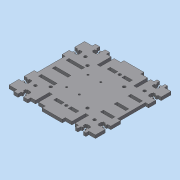
# Autodesk Inventor part: Camera-Holder_Top
Saved by Autodesk Inventor 2016 SP1 (Build 200210100, 210)
## iProperties
Created: 2016-01-28
Part Number: Camera-Holder_Top
Material: Generic
Document SubType Name: Modeling
Designer: Mohamed A.
Density: 1 g/cm^3
Appearance: Default
Author: Mohamed A.
Autodesk Inventor part; units mm, degrees
ref_plane "YZ Plane" through (0, 0, 0) normal (1, 0, 0) x (0, 1, 0)
ref_plane "XZ Plane" through (0, 0, 0) normal (0, 1, 0) x (-1, 0, 0)
ref_plane "XY Plane" through (0, 0, 0) normal (0, 0, 1) x (1, 0, 0)
sketch "Sketch1" plane through (0, 0, 0) normal (0, 0, 1) x (1, 0, 0)
  line L0 (-42.3333, -40) -> (42.3333, -40)
  line L1 (42.3333, -40) -> (42.3333, 40)
  line L2 (42.3333, 40) -> (-42.3333, 40)
  line L3 (-42.3333, 40) -> (-42.3333, -40)
  line L4 (0, 40) -> (0, -40) construction
  line L5 (42.3333, 0) -> (-42.3333, 0) construction
  point P0 (0, 0)
  dimension "d0" = 84.6667
  dimension "d1" = 80
  constraints: 12 end point, 6 midpoint, 2 parallel, 1 horizontal, 1 perpendicular
  measures "d0" distance of L2.end L1.end
  measures "d1" distance of L1.end L0.end
extrude "Extrusion1" add sketch "Sketch1" along normal blind 3
sketch "Sketch2" plane through (-42.3333, 40, 0) normal (0, 1, 0) x (1, 0, 0)
  line L0 (26, -3) -> (26, 0)
  line L1 (26, 0) -> (29, 0)
  line L2 (29, 0) -> (29, -3)
  line L3 (29, -30) -> (26, -30)
  line L4 (0, -3) -> (0, 0)
  line L5 (0, 0) -> (3, 0)
  line L6 (3, 0) -> (3, -3)
  line L7 (3, -30) -> (0, -30)
  line L8 (61.6667, -3) -> (61.6667, 0)
  line L9 (61.6667, 0) -> (64.6667, 0)
  line L10 (64.6667, 0) -> (64.6667, -3)
  line L11 (64.6667, -30) -> (61.6667, -30)
  line L12 (81.6667, -3) -> (81.6667, 0)
  line L13 (81.6667, 0) -> (84.6667, 0)
  line L14 (84.6667, 0) -> (84.6667, -3)
  line L15 (84.6667, -30) -> (81.6667, -30)
  line L16 (84.6667, -3) -> (0, -3) projected
  line L17 (0, -3) -> (3, -3)
  line L18 (26, -3) -> (29, -3)
  line L19 (0, 0) -> (84.6667, 0) projected
  line L20 (3, -3) -> (7.6, -3)
  line L21 (7.6, -3) -> (7.6, 0)
  line L22 (7.6, 0) -> (3, 0)
  line L23 (3, 0) -> (3, -3)
  line L24 (26, -3) -> (21.4, -3)
  line L25 (21.4, -3) -> (21.4, 0)
  line L26 (21.4, 0) -> (26, 0)
  line L27 (26, 0) -> (26, -3)
  line L28 (29, -3) -> (35.5333, -3)
  line L29 (35.5333, -3) -> (35.5333, 0)
  line L30 (35.5333, 0) -> (29, 0)
  line L31 (29, 0) -> (29, -3)
  line L32 (61.6667, -3) -> (55.1333, -3)
  line L33 (55.1333, -3) -> (55.1333, 0)
  line L34 (55.1333, 0) -> (61.6667, 0)
  line L35 (61.6667, 0) -> (61.6667, -3)
  line L36 (64.6667, -3) -> (68.0667, -3)
  line L37 (68.0667, -3) -> (68.0667, 0)
  line L38 (68.0667, 0) -> (64.6667, 0)
  line L39 (64.6667, 0) -> (64.6667, -3)
  line L40 (81.6667, -3) -> (78.2667, -3)
  line L41 (78.2667, -3) -> (78.2667, 0)
  line L42 (78.2667, 0) -> (81.6667, 0)
  line L43 (81.6667, 0) -> (81.6667, -3)
  line L44 (81.6667, -3) -> (84.6667, -3)
  line L45 (64.6667, -3) -> (61.6667, -3)
  line L46 (29, -3) -> (26, -3)
  point P0 (42.3333, 0)
  dimension "d6" = 23
  dimension "d7" = 4.6
  dimension "d8" = 4.6
  dimension "d9" = 17
  dimension "d10" = 3.4
  dimension "d11" = 3.4
  dimension "d12" = 32.6667
  dimension "d34" = 6.5333
  dimension "d35" = 6.5333
  constraints: 90 end point, 14 horizontal, 12 parallel, 8 point on line, 8 vertical, 6 perpendicular, 3 collinear, 23 other
  measures "d6" distance between parallel lines of L23 L27
  measures "d7" distance between parallel lines of L25 L27
  measures "d8" distance between parallel lines of L23 L21
  measures "d9" distance between parallel lines of L10 L12
  measures "d10" distance between parallel lines of L41 L12
  measures "d11" distance between parallel lines of L10 L37
  measures "d12" distance between parallel lines of L31 L8
  measures "d34" distance between parallel lines of L31 L29
  measures "d35" distance between parallel lines of L33 L35
extrude "Extrusion2" cut sketch "Sketch2" against normal blind 3 contours L16 L25 L19 L0 | L0 L1 L2 L16 | L2 L19 L29 L16 | L16 L6 L19 L21 | L33 L19 L8 L16 | L16 L4 L5 L6 | L8 L9 L10 L16 | L10 L19 L37 L16 | L41 L19 L12 L16 | L12 L13 L14 L16
sketch "Sketch3" plane through (-42.3333, -40, 0) normal (0, -1, 0) x (1, 0, 0)
  line L0 (21.4, 3) -> (21.4, 0) projected
  line L1 (35.5333, 0) -> (35.5333, 3) projected
  line L2 (21.4, 0) -> (35.5333, 0) projected
  line L3 (35.5333, 3) -> (21.4, 3) projected
  line L4 (7.6, 0) -> (7.6, 3) projected
  line L5 (0, 0) -> (7.6, 0) projected
  line L6 (0, 3) -> (0, 0) projected
  line L7 (7.6, 3) -> (0, 3) projected
  line L8 (84.6667, 0) -> (84.6667, 3) projected
  line L9 (78.2667, 0) -> (84.6667, 0) projected
  line L10 (78.2667, 3) -> (78.2667, 0) projected
  line L11 (84.6667, 3) -> (78.2667, 3) projected
  line L12 (68.0667, 0) -> (68.0667, 3) projected
  line L13 (55.1333, 0) -> (68.0667, 0) projected
  line L14 (55.1333, 3) -> (55.1333, 0) projected
  line L15 (68.0667, 3) -> (55.1333, 3) projected
  point P0 (42.3333, 0)
extrude "Extrusion3" cut sketch "Sketch3" against normal blind 3
sketch "Sketch5" plane through (0, 0, 0) normal (0, 0, -1) x (-1, 0, 0)
  line L0 (35.5, 14.9948) -> (35.5, 11.9948)
  line L1 (35.5, 11.9948) -> (20.1667, 11.9948)
  line L2 (20.1667, 11.9948) -> (20.1667, 14.9948)
  line L3 (20.1667, 14.9948) -> (35.5, 14.9948)
  line L4 (35.5, -12.0052) -> (35.5, -15.0052)
  line L5 (35.5, -15.0052) -> (20.1667, -15.0052)
  line L6 (20.1667, -15.0052) -> (20.1667, -12.0052)
  line L7 (20.1667, -12.0052) -> (35.5, -12.0052)
  line L8 (35.4997, -1.5) -> (20.1663, -1.5)
  line L9 (20.1663, -1.5) -> (20.1663, 1.5)
  line L10 (20.1663, 1.5) -> (35.4997, 1.5)
  line L11 (35.4997, 1.5) -> (35.4997, -1.5)
  line L12 (-25.1667, -1.5) -> (-36.5, -1.5)
  line L13 (-36.5, -1.5) -> (-36.5, 1.5)
  line L14 (-36.5, 1.5) -> (-25.1667, 1.5)
  line L15 (-25.1667, 1.5) -> (-25.1667, -1.5)
  line L16 (-25.1667, 14.9948) -> (-25.1667, 11.9948)
  line L17 (-25.1667, 11.9948) -> (-36.5, 11.9948)
  line L18 (-36.5, 11.9948) -> (-36.5, 14.9948)
  line L19 (-36.5, 14.9948) -> (-25.1667, 14.9948)
  line L20 (-36.5, -15.0052) -> (-36.5, -12.0052)
  line L21 (-36.5, -12.0052) -> (-25.1667, -12.0052)
  line L22 (-25.1667, -12.0052) -> (-25.1667, -15.0052)
  line L23 (-25.1667, -15.0052) -> (-36.5, -15.0052)
  line L24 (-39.3333, -12.3333) -> (-39.3333, 14.9948)
  line L25 (-39.3333, 14.9948) -> (-42.3333, 14.9948)
  line L26 (-42.3333, -37) -> (-42.3333, 37) projected
  line L27 (-39.3333, -12.3333) -> (-42.3333, -12.3333)
  line L28 (0, -54.8385) -> (0, 51.4251) construction
  line L29 (39.3333, -12.3333) -> (39.3333, 14.9948)
  line L30 (39.3333, 14.9948) -> (42.3333, 14.9948)
  line L31 (39.3333, -12.3333) -> (42.3333, -12.3333)
  line L32 (-42.3333, -22.0167) -> (-39.3333, -22.0167)
  line L33 (-39.3333, -22.0167) -> (-39.3333, -23.1667)
  line L34 (-39.3333, -23.1667) -> (-37.3333, -23.1667)
  line L35 (-37.3333, -23.1667) -> (-37.3333, -22.0167)
  line L36 (-37.3333, -22.0167) -> (-34.9333, -22.0167)
  line L37 (-34.9333, -22.0167) -> (-34.9333, -23.1667)
  line L38 (-34.9333, -23.1667) -> (-34.3333, -23.1667)
  line L39 (-34.3333, -23.1667) -> (-34.3333, -26.1667)
  line L40 (-34.3333, -26.1667) -> (-34.9333, -26.1667)
  line L41 (-34.9333, -26.1667) -> (-34.9333, -27.3167)
  line L42 (-34.9333, -27.3167) -> (-37.3333, -27.3167)
  line L43 (-37.3333, -27.3167) -> (-37.3333, -26.1667)
  line L44 (-39.3333, -26.1667) -> (-37.3333, -26.1667)
  line L45 (-39.3333, -26.1667) -> (-39.3333, -27.3167)
  line L46 (-39.3333, -27.3167) -> (-42.3333, -27.3167)
  line L47 (-42.3333, -24.6667) -> (-30.9977, -24.6667) construction
  line L48 (-42.3333, -37) -> (-35.9333, -37) construction
  line L49 (60.8093, 0) -> (-56.5226, 0) construction
  line L50 (-42.3333, 22.0167) -> (-39.3333, 22.0167)
  line L51 (-39.3333, 22.0167) -> (-39.3333, 23.1667)
  line L52 (-39.3333, 23.1667) -> (-37.3333, 23.1667)
  line L53 (-37.3333, 23.1667) -> (-37.3333, 22.0167)
  line L54 (-37.3333, 22.0167) -> (-34.9333, 22.0167)
  line L55 (-34.9333, 22.0167) -> (-34.9333, 23.1667)
  line L56 (-34.9333, 23.1667) -> (-34.3333, 23.1667)
  line L57 (-34.3333, 23.1667) -> (-34.3333, 26.1667)
  line L58 (-34.3333, 26.1667) -> (-34.9333, 26.1667)
  line L59 (-34.9333, 26.1667) -> (-34.9333, 27.3167)
  line L60 (-34.9333, 27.3167) -> (-37.3333, 27.3167)
  line L61 (-37.3333, 27.3167) -> (-37.3333, 26.1667)
  line L62 (-39.3333, 26.1667) -> (-37.3333, 26.1667)
  line L63 (-39.3333, 26.1667) -> (-39.3333, 27.3167)
  line L64 (-39.3333, 27.3167) -> (-42.3333, 27.3167)
  line L65 (42.3333, -22.0167) -> (39.3333, -22.0167)
  line L66 (39.3333, -22.0167) -> (39.3333, -23.1667)
  line L67 (39.3333, -23.1667) -> (37.3333, -23.1667)
  line L68 (37.3333, -23.1667) -> (37.3333, -22.0167)
  line L69 (37.3333, -22.0167) -> (34.9333, -22.0167)
  line L70 (34.9333, -22.0167) -> (34.9333, -23.1667)
  line L71 (34.9333, -23.1667) -> (34.3333, -23.1667)
  line L72 (34.3333, -23.1667) -> (34.3333, -26.1667)
  line L73 (34.3333, -26.1667) -> (34.9333, -26.1667)
  line L74 (34.9333, -26.1667) -> (34.9333, -27.3167)
  line L75 (34.9333, -27.3167) -> (37.3333, -27.3167)
  line L76 (37.3333, -27.3167) -> (37.3333, -26.1667)
  line L77 (39.3333, -26.1667) -> (37.3333, -26.1667)
  line L78 (39.3333, -26.1667) -> (39.3333, -27.3167)
  line L79 (39.3333, -27.3167) -> (42.3333, -27.3167)
  line L80 (34.3333, 23.1667) -> (34.3333, 26.1667)
  line L81 (34.9333, 23.1667) -> (34.3333, 23.1667)
  line L82 (34.9333, 22.0167) -> (34.9333, 23.1667)
  line L83 (37.3333, 22.0167) -> (34.9333, 22.0167)
  line L84 (37.3333, 23.1667) -> (37.3333, 22.0167)
  line L85 (39.3333, 23.1667) -> (37.3333, 23.1667)
  line L86 (39.3333, 22.0167) -> (39.3333, 23.1667)
  line L87 (42.3333, 22.0167) -> (39.3333, 22.0167)
  line L88 (39.3333, 27.3167) -> (42.3333, 27.3167)
  line L89 (39.3333, 26.1667) -> (39.3333, 27.3167)
  line L90 (39.3333, 26.1667) -> (37.3333, 26.1667)
  line L91 (37.3333, 27.3167) -> (37.3333, 26.1667)
  line L92 (34.9333, 27.3167) -> (37.3333, 27.3167)
  line L93 (34.9333, 26.1667) -> (34.9333, 27.3167)
  line L94 (34.3333, 26.1667) -> (34.9333, 26.1667)
  line L95 (-42.3333, 37) -> (-42.3333, -37) projected
  line L96 (-42.3333, 27.3167) -> (-42.3333, 22.0167)
  line L97 (42.3333, 27.3167) -> (42.3333, 22.0167)
  line L98 (42.3333, 37) -> (42.3333, -37) projected
  line L99 (42.3333, -22.0167) -> (42.3333, -27.3167)
  line L100 (42.3333, 14.9948) -> (42.3333, -12.3333)
  line L101 (-35.9333, 40) -> (-25.7333, 40) construction
  line L102 (-30.8333, 40) -> (-30.8333, 25.5661) construction
  line L103 (-33.4833, 40) -> (-28.1833, 40)
  line L104 (-28.1833, 37) -> (-28.1833, 40)
  line L105 (-28.1833, 37) -> (-29.3333, 37)
  line L106 (-29.3333, 37) -> (-29.3333, 35)
  line L107 (-29.3333, 35) -> (-28.1833, 35)
  line L108 (-28.1833, 35) -> (-28.1833, 32.6)
  line L109 (-28.1833, 32.6) -> (-29.3333, 32.6)
  line L110 (-29.3333, 32.6) -> (-29.3333, 32)
  line L111 (-29.3333, 32) -> (-32.3333, 32)
  line L112 (-32.3333, 32) -> (-32.3333, 32.6)
  line L113 (-32.3333, 32.6) -> (-33.4833, 32.6)
  line L114 (-33.4833, 32.6) -> (-33.4833, 35)
  line L115 (-33.4833, 35) -> (-32.3333, 35)
  line L116 (-32.3333, 37) -> (-33.4833, 37)
  line L117 (-33.4833, 40) -> (-33.4833, 37)
  line L118 (-32.3333, 37) -> (-32.3333, 35)
  line L119 (-33.4833, -40) -> (-28.1833, -40)
  line L120 (-28.1833, -37) -> (-28.1833, -40)
  line L121 (-28.1833, -37) -> (-29.3333, -37)
  line L122 (-29.3333, -37) -> (-29.3333, -35)
  line L123 (-29.3333, -35) -> (-28.1833, -35)
  line L124 (-28.1833, -35) -> (-28.1833, -32.6)
  line L125 (-28.1833, -32.6) -> (-29.3333, -32.6)
  line L126 (-29.3333, -32.6) -> (-29.3333, -32)
  line L127 (-29.3333, -32) -> (-32.3333, -32)
  line L128 (-32.3333, -32) -> (-32.3333, -32.6)
  line L129 (-32.3333, -32.6) -> (-33.4833, -32.6)
  line L130 (-33.4833, -32.6) -> (-33.4833, -35)
  line L131 (-33.4833, -35) -> (-32.3333, -35)
  line L132 (-32.3333, -37) -> (-33.4833, -37)
  line L133 (-33.4833, -40) -> (-33.4833, -37)
  line L134 (-32.3333, -37) -> (-32.3333, -35)
  line L135 (27.8333, 40.9143) -> (27.8333, 27.3377) construction
  line L136 (25.1833, 40) -> (30.4833, 40)
  line L137 (30.4833, 37) -> (30.4833, 40)
  line L138 (30.4833, 37) -> (29.3333, 37)
  line L139 (29.3333, 37) -> (29.3333, 35)
  line L140 (29.3333, 35) -> (30.4833, 35)
  line L141 (30.4833, 35) -> (30.4833, 32.6)
  line L142 (30.4833, 32.6) -> (29.3333, 32.6)
  line L143 (29.3333, 32.6) -> (29.3333, 32)
  line L144 (29.3333, 32) -> (26.3333, 32)
  line L145 (26.3333, 32) -> (26.3333, 32.6)
  line L146 (26.3333, 32.6) -> (25.1833, 32.6)
  line L147 (25.1833, 32.6) -> (25.1833, 35)
  line L148 (25.1833, 35) -> (26.3333, 35)
  line L149 (26.3333, 37) -> (25.1833, 37)
  line L150 (25.1833, 40) -> (25.1833, 37)
  line L151 (26.3333, 37) -> (26.3333, 35)
  line L152 (34.7333, 40) -> (20.9333, 40) projected
  line L153 (20.9333, 40) -> (20.9333, 37) projected
  line L154 (34.7333, 37) -> (34.7333, 40) projected
  line L155 (30.4833, -37) -> (30.4833, -40)
  line L156 (25.1833, -40) -> (30.4833, -40)
  line L157 (25.1833, -40) -> (25.1833, -37)
  line L158 (26.3333, -37) -> (25.1833, -37)
  line L159 (26.3333, -37) -> (26.3333, -35)
  line L160 (25.1833, -35) -> (26.3333, -35)
  line L161 (25.1833, -32.6) -> (25.1833, -35)
  line L162 (26.3333, -32.6) -> (25.1833, -32.6)
  line L163 (26.3333, -32) -> (26.3333, -32.6)
  line L164 (29.3333, -32) -> (26.3333, -32)
  line L165 (29.3333, -32.6) -> (29.3333, -32)
  line L166 (30.4833, -32.6) -> (29.3333, -32.6)
  line L167 (30.4833, -35) -> (30.4833, -32.6)
  line L168 (29.3333, -35) -> (30.4833, -35)
  line L169 (29.3333, -37) -> (29.3333, -35)
  line L170 (30.4833, -37) -> (29.3333, -37)
  line L171 (-19.3333, 23.4685) -> (-22.3333, 23.4685)
  line L172 (-22.3333, 23.4685) -> (-22.3333, 40)
  line L173 (-22.3333, 40) -> (-19.3333, 40)
  line L174 (-19.3333, 40) -> (-19.3333, 23.4685)
  line L175 (-19.3333, -40) -> (-22.3333, -40)
  line L176 (-22.3333, -40) -> (-22.3333, -23.5315)
  line L177 (-22.3333, -23.5315) -> (-19.3333, -23.5315)
  line L178 (-19.3333, -23.5315) -> (-19.3333, -40)
  line L179 (16.3333, 23.4685) -> (13.3333, 23.4685)
  line L180 (13.3333, 23.4685) -> (13.3333, 40)
  line L181 (13.3333, 40) -> (16.3333, 40)
  line L182 (16.3333, 40) -> (16.3333, 23.4685)
  line L183 (16.3333, -40) -> (13.3333, -40)
  line L184 (13.3333, -40) -> (13.3333, -23.5315)
  line L185 (13.3333, -23.5315) -> (16.3333, -23.5315)
  line L186 (16.3333, -23.5315) -> (16.3333, -40)
  circle A0 centre (-15.5586, 17.9685) radius 1.5 construction
  circle A1 centre (20.4414, 17.9685) radius 1.5 construction
  circle A2 centre (20.4414, -18.0315) radius 1.5 construction
  circle A3 centre (-15.5586, -18.0315) radius 1.5 construction
  circle A4 centre (20.4414, 17.9685) radius 1.4
  circle A5 centre (20.4414, -18.0315) radius 1.4
  circle A6 centre (-15.5586, -18.0315) radius 1.4
  circle A7 centre (-15.5586, 17.9685) radius 1.4
  line L187 (-29, -24.5) -> (29, -24.5) construction
  line L188 (29, -24.5) -> (29, 24.5) construction
  line L189 (29, 24.5) -> (-29, 24.5) construction
  line L190 (-29, 24.5) -> (-29, -24.5) construction
  line L191 (-29, -24.5) -> (29, 24.5) construction
  line L192 (29, -24.5) -> (-29, 24.5) construction
  circle A8 centre (29, 24.5) radius 1.4
  circle A9 centre (-29, 24.5) radius 1.4
  circle A10 centre (-29, -24.5) radius 1.4
  circle A11 centre (29, -24.5) radius 1.4
  line L193 (-13.8889, 27.6685) -> (-6.5, 27.6685) projected
  line L194 (-6.5, 27.6685) -> (-6.5, 24.6685) projected
  line L195 (-13.8889, 24.6685) -> (-6.5, 24.6685) projected
  line L196 (-13.8889, 27.6685) -> (-13.8889, 24.6685) projected
  line L197 (0.5, 27.6685) -> (7.8889, 27.6685) projected
  line L198 (7.8889, 27.6685) -> (7.8889, 24.6685) projected
  line L199 (0.5, 24.6685) -> (7.8889, 24.6685) projected
  line L200 (0.5, 27.6685) -> (0.5, 24.6685) projected
  line L201 (0.5, -24.7315) -> (7.8889, -24.7315) projected
  line L202 (7.8889, -24.7315) -> (7.8889, -27.7315) projected
  line L203 (0.5, -27.7315) -> (7.8889, -27.7315) projected
  line L204 (0.5, -24.7315) -> (0.5, -27.7315) projected
  line L205 (-13.8889, -24.7315) -> (-6.5, -24.7315) projected
  line L206 (-6.5, -24.7315) -> (-6.5, -27.7315) projected
  line L207 (-13.8889, -27.7315) -> (-6.5, -27.7315) projected
  line L208 (-13.8889, -24.7315) -> (-13.8889, -27.7315) projected
  line L209 (0.5, -27.7315) -> (-6.5, -24.7315) construction
  line L210 (-6.5, -27.7315) -> (0.5, -24.7315) construction
  circle A12 centre (-3, -26.2315) radius 1.35
  line L211 (0.5, 24.6685) -> (-6.5, 27.6685) construction
  line L212 (-6.5, 24.6685) -> (0.5, 27.6685) construction
  circle A13 centre (-3, 26.1685) radius 1.35
  circle A14 centre (-0.1086, -10.5315) radius 0.9 projected
  circle A15 centre (12.3914, -10.5315) radius 0.9 projected
  circle A16 centre (12.3914, 10.4685) radius 0.9 projected
  circle A17 centre (-0.1086, 10.4685) radius 0.9 projected
  point P0 (0, 0)
  dimension "d24" = 3
  dimension "d25" = 5.3
  dimension "d26" = 3
  dimension "d27" = 2.4
  dimension "d28" = 8
  dimension "d30" = 12.3333
  dimension "d31" = 5
  dimension "d32" = 37
  dimension "d33" = 24.6667
  dimension "d36" = 3
  dimension "d37" = 5.3
  dimension "d38" = 2.4
  dimension "d39" = 3
  dimension "d40" = 8
  dimension "d41" = 5
  dimension "d42" = 3
  dimension "d43" = 5.3
  dimension "d44" = 2.4
  dimension "d45" = 3
  dimension "d46" = 8
  dimension "d47" = 5
  dimension "d48" = 13.8
  dimension "d49" = 6.9
  dimension "d50" = 2.8
  dimension "d51" = 2.8
  dimension "d52" = 2.8
  dimension "d53" = 2.8
  dimension "d54" = 58
  dimension "d55" = 49
  dimension "d56" = 2.8
  dimension "d57" = 2.8
  dimension "d58" = 2.8
  dimension "d59" = 2.8
  dimension "d60" = 2.7
  dimension "d61" = 2.7
  constraints: 378 end point, 119 point on line, 84 symmetric about line, 29 perpendicular, 28 horizontal, 26 vertical, 14 centre point, 8 coincident, 5 collinear, 5 midpoint, 3 parallel, 54 other
  measures "d24" distance of L24.start L27.end
  measures "d25" distance between parallel lines of L32 L46
  measures "d26" distance between parallel lines of L34 L44
  measures "d27" distance between parallel lines of L43 L41
  measures "d28" distance between parallel lines of L26 L39
  measures "d30" distance between parallel lines of L47 L48
  measures "d31" distance between parallel lines of L26 L43
  measures "d32" distance between parallel lines of L49 L48
  measures "d33" distance between parallel lines of L27 L48
  measures "d36" distance between parallel lines of L118 L106
  measures "d37" distance between parallel lines of L114 L108
  measures "d38" distance between parallel lines of L109 L107
  measures "d39" distance between parallel lines of L103 L105
  measures "d40" distance between parallel lines of L103 L111
  measures "d41" distance between parallel lines of L103 L107
  measures "d42" distance between parallel lines of L151 L139
  measures "d43" distance between parallel lines of L147 L141
  measures "d44" distance between parallel lines of L142 L140
  measures "d45" distance between parallel lines of L136 L138
  measures "d46" distance between parallel lines of L136 L144
  measures "d47" distance between parallel lines of L136 L140
  measures "d48" distance between parallel lines of L153 L154
  measures "d49" distance between parallel lines of L135 L154
  measures "d50" diameter of A4
  measures "d51" diameter of A5
  measures "d52" diameter of A6
  measures "d53" diameter of A7
  measures "d54" distance of L189.end L188.end
  measures "d55" distance of L188.end L187.end
  measures "d56" diameter of A8
  measures "d57" diameter of A9
  measures "d58" diameter of A10
  measures "d59" diameter of A11
  measures "d60" diameter of A12
  measures "d61" diameter of A13
extrude "Extrusion5" cut sketch "Sketch5" against normal blind 3
equation "\"d7\" = d8"
equation "\"d8\" = 0.2 * d6"
equation "\"d10\" = 0.2 * d9"
equation "\"d11\" = d10"
equation "\"d34\" = 0.2 * d12"
equation "\"d35\" = d34"
equation "\"d30\" = 0.5 * d33"
equation "\"d33\" = 0.666667 * d32"
equation "\"d49\" = 0.5 * d48"
body "Solid1"
